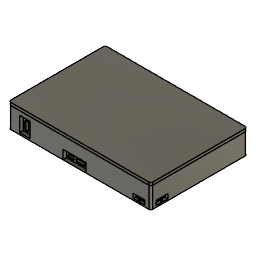
CXD_ROUTER (Autodesk Fusion 360 design; units mm, degrees)
Autodesk Fusion 360 part; units mm, degrees
sketch "Sketch1" plane through (0, 0, 0) normal (0, 0, 1) x (1, 0, 0)
  line L0 (0, 0) -> (150, 0)
  line L1 (150, 0) -> (150, 100)
  line L2 (150, 100) -> (0, 100)
  line L3 (0, 100) -> (0, 0)
  dimension "d1" = 150
  dimension "d2" = 100
  constraint horizontal L0
  constraint vertical L1
  constraint horizontal L2
  constraint vertical L3
  constraint coincident L0.start L3.end
  measures "d1" distance of L0.start L0.end
  measures "d2" distance of L0.start L2.end
extrude "Extrude1" add sketch "Sketch1" along normal blind 3 makes body 1
shell "Shell1" thickness 3 outward yes removed faces 1 at (50, 66.6667, 3) on bodies 1
extrude "Extrude2" add 1 faces at (100, -2, 3) along direction (0, 0, 1) blind 2 on bodies 1 bodies 1
extrude "Extrude3" add 1 faces at (100, -2, 5) along direction (0, 0, 1) blind 5 on bodies 1 bodies 1
extrude "Extrude4" add 1 faces at (100, -2, 10) along direction (0, 0, 1) blind 10 on bodies 1 bodies 1
sketch "Sketch2" plane through (0, 0, 20) normal (0, 0, 1) x (-1, 0, 0)
  line L0 (0, -100) -> (-150, -100)
  line L1 (-150, -100) -> (-150, 0)
  line L2 (-150, 0) -> (0, 0)
  line L3 (0, 0) -> (0, -100)
  line L4 (3, -103) -> (3, 3)
  line L5 (3, 3) -> (-153, 3)
  line L6 (-153, 3) -> (-153, -103)
  line L7 (-153, -103) -> (3, -103)
  line L8 (3, -103) -> (-153, -103)
  line L9 (-153, -103) -> (-153, 3)
  line L10 (-153, 3) -> (3, 3)
  line L11 (3, 3) -> (3, -103)
  constraint horizontal L8
  constraint vertical L9
  constraint horizontal L10
  constraint vertical L11
  constraint coincident L5.end L6.start
  constraint coincident L4.start L7.end
extrude "Extrude5" add sketch "Sketch2" along normal blind 3 separate body contours L0 L1 L2 L3 | L4 L5 L6 L7 L8 L9 L10 L11 makes body 2
other "Base Mesh Feature1"
sketch "Sketch3" plane through (0, 0, 0) normal (0, 1, 0) x (-1, 0, 0)
  line L0 (-150, 0) -> (0, 0)
  line L1 (0, 0) -> (0, 20)
  line L2 (0, 20) -> (-150, 20)
  line L3 (-150, 20) -> (-150, 0)
  line L4 (-16.6, 2.5) -> (-12.9425, 2.5)
  line L5 (-12.9425, 2.5) -> (-12.9425, 11.8)
  line L6 (-12.9425, 11.8) -> (-16.5, 11.8)
  line L7 (-16.6, 2.5) -> (-16.6, 11.8)
  line L8 (-16.6, 11.8) -> (-16.5, 11.8)
  constraint horizontal L4
  constraint perpendicular L4 L5
  constraint perpendicular L5 L6
  constraint perpendicular L4 L7
  constraint perpendicular L7 L8
extrude "Extrude6" cut sketch "Sketch3" against normal blind 9 contours L4 L5 L6 L7 L8 bodies 1
sketch "Sketch4" plane through (0, 0, 0) normal (0, 1, 0) x (-1, 0, 0)
  line L0 (-61.2, 0.3) -> (-66.1, 0.3)
  line L1 (-66.1, 0.3) -> (-66.9, 1.1)
  line L2 (-66.9, 1.1) -> (-66.9, 3.4)
  line L3 (-66.9, 3.4) -> (-60.3, 3.4)
  line L4 (-60.3, 3.4) -> (-60.3, 1.1)
  line L5 (-60.3, 1.1) -> (-61.2, 0.3)
  line L6 (-77.3, 0.3) -> (-69.3, 0.3)
  line L7 (-69.3, 0.3) -> (-69.3, 3.7)
  line L8 (-69.3, 3.7) -> (-78.2, 3.7)
  line L9 (-78.2, 3.7) -> (-78.3, 3.7)
  line L10 (-78.3, 3.7) -> (-78.3, 0.3)
  line L11 (-78.3, 0.3) -> (-77.3, 0.3)
  constraint horizontal L0
  constraint perpendicular L0 L2
  constraint perpendicular L2 L3
  constraint perpendicular L3 L4
  constraint horizontal L6
  constraint perpendicular L6 L7
  constraint perpendicular L7 L8
  constraint perpendicular L7 L9
  constraint perpendicular L9 L10
  constraint perpendicular L10 L11
extrude "Extrude7" cut sketch "Sketch4" against normal blind 16 bodies 1
sketch "Sketch5" plane through (0, -3, 0) normal (0, -1, 0) x (1, 0, 0)
  line L0 (69.3, 0.3) -> (69.3, 3.7)
  line L1 (69.3, 3.7) -> (78.3, 3.7)
  line L2 (78.3, 3.7) -> (78.3, 0.3)
  line L3 (78.3, 0.3) -> (69.3, 0.3)
  line L4 (60.3, 3.4) -> (66.9, 3.4)
  line L5 (66.9, 3.4) -> (66.9, 1.1)
  line L6 (66.9, 1.1) -> (66.1, 0.3)
  line L7 (66.1, 0.3) -> (61.2, 0.3)
  line L8 (61.2, 0.3) -> (60.3, 1.1)
  line L9 (60.3, 1.1) -> (60.3, 3.4)
  line L10 (12.9425, 2.5) -> (12.9425, 11.8)
  line L11 (12.9425, 11.8) -> (16.6, 11.8)
  line L12 (16.6, 11.8) -> (16.6, 2.5)
  line L13 (16.6, 2.5) -> (12.9425, 2.5)
  line L14 (-3, -3) -> (153, -3)
  line L15 (153, -3) -> (153, 20)
  line L16 (153, 20) -> (-3, 20)
  line L17 (-3, 20) -> (-3, -3)
  line L18 (135, 2.2) -> (139.3, 2.2)
  line L19 (139.3, 2.2) -> (139.3, 0.3)
  line L20 (139.3, 0.3) -> (135, 0.3)
  line L21 (135, 0.3) -> (135, 2.2)
  line L22 (140.6, 2.2) -> (144.9, 2.2)
  line L23 (144.9, 2.2) -> (144.9, 0.3)
  line L24 (144.9, 0.3) -> (140.6, 0.3)
  line L25 (140.6, 0.3) -> (140.6, 2.2)
  constraint horizontal L18
  constraint vertical L19
  constraint horizontal L20
  constraint vertical L21
  constraint horizontal L22
  constraint vertical L23
  constraint horizontal L24
  constraint vertical L25
extrude "Extrude8" cut sketch "Sketch5" against normal blind 4.5 contours L18 L19 L20 L21 | L22 L23 L24 L25 bodies 1
sketch "Sketch6" plane through (153, 0, 0) normal (1, 0, 0) x (0, 1, 0)
  line L0 (-3, -3) -> (103, -3)
  line L1 (103, -3) -> (103, 20)
  line L2 (103, 20) -> (-3, 20)
  line L3 (-3, 20) -> (-3, -3)
  line L4 (8.8, 0.3) -> (4.5193, 0.3)
  line L5 (4.5193, 0.3) -> (4.5193, 2.1512)
  line L6 (4.5193, 2.1512) -> (8.8, 2.1512)
  line L7 (8.8, 2.1512) -> (8.8, 0.3)
  line L8 (10.2, 0.3) -> (14.4, 0.3)
  line L9 (14.4, 0.3) -> (14.4, 2.1)
  line L10 (14.4, 2.1) -> (10.2, 2.1)
  line L11 (10.2, 2.1) -> (10.2, 0.3)
  constraint horizontal L4
  constraint vertical L5
  constraint horizontal L6
  constraint vertical L7
  constraint horizontal L8
  constraint vertical L9
  constraint horizontal L10
  constraint vertical L11
extrude "Extrude9" cut sketch "Sketch6" against normal blind 16 contours L4 L5 L6 L7 | L8 L9 L10 L11 bodies 1
chamfer "Chamfer1" distance 1.5 angle 45 8 edges at (142.75, -3, 0.3) (137.15, -3, 0.3) (137.15, -3, 2.2) (142.75, -3, 2.2) (153, 6.6597, 0.3) (153, 12.3, 0.3) (153, 12.3, 2.1) (153, 6.6597, 2.1512) on bodies 1
chamfer "Chamfer2" distance 1.5 angle 45 4 edges at (153, 14.4, 1.2) (153, 4.5193, 1.2256) (144.9, -3, 1.25) (135, -3, 1.25) on bodies 1
chamfer "Chamfer3" distance 0.5 angle 45 4 edges at (153, 8.8, 1.2256) (153, 10.2, 1.2) (139.3, -3, 1.25) (140.6, -3, 1.25) on bodies 1
extrude "Extrude10" cut 1 faces at (15.3808, -1, 2.5) along direction (0, 0, -1) blind 0.2 on bodies 1 bodies 1
extrude "Extrude11" cut 1 faces at (12.9425, -1, 5.4667) along direction (-1, 0, 0) blind 0.2 on bodies 1 bodies 1
extrude "Extrude12" cut 1 faces at (16.6, -1, 8.6333) along direction (1, 0, 0) blind 0.2 on bodies 1 bodies 1
extrude "Extrude13" cut 1 faces at (14.095, -1, 11.8) along direction (0, 0, 1) blind 0.2 on bodies 1 bodies 1
extrude "Extrude14" cut 1 faces at (72.3, -1, 3.7) along direction (0, 0, 1) blind 0.2 on bodies 1 bodies 1
extrude "Extrude15" cut 1 faces at (64.7, -1, 3.4) along direction (0, 0, 1) blind 0.2 on bodies 1 bodies 1
fillet "Fillet1" radius 1 4 edges at (12.7425, -1.5, 2.3) (12.7425, -1.5, 12) (16.8, -1.5, 12) (16.8, -1.5, 2.3) on bodies 1
extrude "Extrude16" cut 1 faces at (78.3, -1, 2.7) along direction (1, 0, 0) blind 0.2 on bodies 1 bodies 1
extrude "Extrude17" cut 1 faces at (69.3, -1, 1.5) along direction (-1, 0, 0) blind 0.2 on bodies 1 bodies 1
fillet "Fillet2" radius 1 4 edges at (69.1, -1.5, 3.9) (78.5, -1.5, 0.3) (78.5, -1.5, 3.9) (69.1, -1.5, 0.3) on bodies 1
fillet "Fillet3" radius 1 6 edges at (60.3, -1.5, 3.6) (66.9, -1.5, 1.1) (66.1, -1.5, 0.3) (60.3, -1.5, 1.1) (61.2, -1.5, 0.3) (66.9, -1.5, 3.6) on bodies 1
sketch "Sketch7" plane through (0, 0, 20) normal (0, 0, 1) x (-1, 0, 0)
  line L0 (0, -100) -> (-150, -100)
  line L1 (-150, -100) -> (-150, 0)
  line L2 (-150, 0) -> (0, 0)
  line L3 (0, 0) -> (0, -100)
  line L4 (3, -103) -> (3, 3)
  line L5 (3, 3) -> (-153, 3)
  line L6 (-153, 3) -> (-153, -103)
  line L7 (-153, -103) -> (3, -103)
  line L8 (-90, -76) -> (-69, -76)
  line L9 (-69, -76) -> (-69, -99)
  line L10 (-69, -99) -> (-90, -99)
  line L11 (-90, -99) -> (-90, -76)
  constraint horizontal L8
  constraint vertical L9
  constraint horizontal L10
  constraint vertical L11
extrude "Extrude18" add sketch "Sketch7" against normal blind 20 separate body contours L8 L9 L10 L11 makes body 3
extrude "Extrude19" cut 1 faces at (83, 83.6667, 20) along direction (0, 0, -1) blind 3 on bodies 3 bodies 3
extrude "Extrude20" cut 1 faces at (76, 99, 5.6667) along direction (0, 1, 0) blind 6 on bodies 3 bodies 1
fillet "Fillet4" radius 1 4 edges at (90, 101.5, 0) (69, 101.5, 0) (69, 101.5, 17) (90, 101.5, 17) on bodies 1
fillet "Fillet5" radius 2 4 edges at (-3, 103, 8.5) (153, 103, 8.5) (-3, -3, 8.5) (153, -3, 8.5) on bodies 1
fillet "Fillet6" radius 2 4 edges at (153, -3, 21.5) (153, 103, 21.5) (-3, 103, 21.5) (-3, -3, 21.5) on bodies 2
sketch "Sketch8" plane through (0, -3, 0) normal (0, -1, 0) x (1, 0, 0)
  line L0 (139.8, -1.2) -> (133.5, -1.2)
  line L1 (133.5, -1.2) -> (133.5, 3.7)
  line L2 (133.5, 3.7) -> (139.8, 3.7)
  line L3 (139.8, 3.7) -> (139.8, -1.2)
  line L4 (140.1, 3.7) -> (146.4, 3.7)
  line L5 (146.4, 3.7) -> (146.4, -1.2)
  line L6 (146.4, -1.2) -> (140.1, -1.2)
  line L7 (140.1, -1.2) -> (140.1, 3.7)
  line L8 (16.8, 11) -> (16.8, 3.3)
  arc A0 (15.8, 2.3) -> (16.8, 3.3) centre (15.8, 3.3) ccw
  line L9 (15.8, 2.3) -> (13.7425, 2.3)
  arc A1 (12.7425, 3.3) -> (13.7425, 2.3) centre (13.7425, 3.3) ccw
  line L10 (12.7425, 3.3) -> (12.7425, 11)
  arc A2 (13.7425, 12) -> (12.7425, 11) centre (13.7425, 11) ccw
  line L11 (13.7425, 12) -> (15.8, 12)
  arc A3 (16.8, 11) -> (15.8, 12) centre (15.8, 11) ccw
  line L12 (66.9, 2.6) -> (66.9, 1.5142)
  arc A4 (66.6071, 0.8071) -> (66.9, 1.5142) centre (65.9, 1.5142) ccw
  line L13 (66.6071, 0.8071) -> (66.3929, 0.5929)
  arc A5 (65.6858, 0.3) -> (66.3929, 0.5929) centre (65.6858, 1.3) ccw
  line L14 (65.6858, 0.3) -> (61.5802, 0.3)
  arc A6 (60.9158, 0.5526) -> (61.5802, 0.3) centre (61.5802, 1.3) ccw
  line L15 (60.9158, 0.5526) -> (60.6356, 0.8017)
  arc A7 (60.3, 1.5491) -> (60.6356, 0.8017) centre (61.3, 1.5491) ccw
  line L16 (60.3, 1.5491) -> (60.3, 2.6)
  arc A8 (61.3, 3.6) -> (60.3, 2.6) centre (61.3, 2.6) ccw
  line L17 (61.3, 3.6) -> (65.9, 3.6)
  arc A9 (66.9, 2.6) -> (65.9, 3.6) centre (65.9, 2.6) ccw
  line L18 (70.1, 3.9) -> (77.5, 3.9)
  arc A10 (78.5, 2.9) -> (77.5, 3.9) centre (77.5, 2.9) ccw
  line L19 (78.5, 2.9) -> (78.5, 1.3)
  arc A11 (77.5, 0.3) -> (78.5, 1.3) centre (77.5, 1.3) ccw
  line L20 (77.5, 0.3) -> (70.1, 0.3)
  arc A12 (69.1, 1.3) -> (70.1, 0.3) centre (70.1, 1.3) ccw
  line L21 (69.1, 1.3) -> (69.1, 2.9)
  arc A13 (70.1, 3.9) -> (69.1, 2.9) centre (70.1, 2.9) ccw
  line L22 (151, -3) -> (151, 20)
  line L23 (151, 20) -> (-1, 20)
  line L24 (-1, 20) -> (-1, -3)
  line L25 (-1, -3) -> (151, -3)
  line L26 (58.5, 5) -> (80, 5)
  line L27 (80, 5) -> (80, -1)
  line L28 (80, -1) -> (58.5, -1)
  line L29 (58.5, -1) -> (58.5, 5)
  constraint parallel L17 L26
  constraint perpendicular L17 L27
  constraint perpendicular L27 L28
  constraint perpendicular L26 L29
extrude "Extrude21" cut sketch "Sketch8" against normal blind 2 contours L26 L27 L28 L29 bodies 1
sketch "Sketch9" plane through (0, -3, 0) normal (0, -1, 0) x (1, 0, 0)
  line L0 (80, 5) -> (80, -1)
  line L1 (80, -1) -> (58.5, -1)
  line L2 (58.5, -1) -> (58.5, 5)
  line L3 (58.5, 5) -> (80, 5)
  line L4 (139.8, -1.2) -> (133.5, -1.2)
  line L5 (133.5, -1.2) -> (133.5, 3.7)
  line L6 (133.5, 3.7) -> (139.8, 3.7)
  line L7 (139.8, 3.7) -> (139.8, -1.2)
  line L8 (140.1, 3.7) -> (146.4, 3.7)
  line L9 (146.4, 3.7) -> (146.4, -1.2)
  line L10 (146.4, -1.2) -> (140.1, -1.2)
  line L11 (140.1, -1.2) -> (140.1, 3.7)
  line L12 (16.8, 11) -> (16.8, 3.3)
  arc A0 (15.8, 2.3) -> (16.8, 3.3) centre (15.8, 3.3) ccw
  line L13 (15.8, 2.3) -> (13.7425, 2.3)
  arc A1 (12.7425, 3.3) -> (13.7425, 2.3) centre (13.7425, 3.3) ccw
  line L14 (12.7425, 3.3) -> (12.7425, 11)
  arc A2 (13.7425, 12) -> (12.7425, 11) centre (13.7425, 11) ccw
  line L15 (13.7425, 12) -> (15.8, 12)
  arc A3 (16.8, 11) -> (15.8, 12) centre (15.8, 11) ccw
  line L16 (151, -3) -> (151, 20)
  line L17 (151, 20) -> (-1, 20)
  line L18 (-1, 20) -> (-1, -3)
  line L19 (-1, -3) -> (151, -3)
  line L20 (11, 13.5) -> (18.5, 13.5)
  line L21 (18.5, 13.5) -> (18.5, 1)
  line L22 (18.5, 1) -> (11, 1)
  line L23 (11, 1) -> (11, 13.5)
  constraint horizontal L20
  constraint vertical L21
  constraint horizontal L22
  constraint vertical L23
extrude "Extrude22" cut sketch "Sketch9" against normal blind 2 contours L20 L21 L22 L23 bodies 1
chamfer "Chamfer4" distance 2 angle 45 8 edges at (14.75, -3, 13.5) (11, -3, 7.25) (18.5, -3, 7.25) (14.75, -3, 1) (69.25, -3, -1) (58.5, -3, 2) (69.25, -3, 5) (80, -3, 2) on bodies 1
hidden bodies 3
